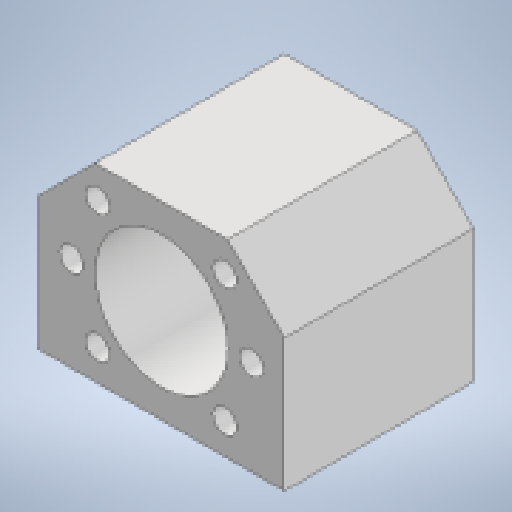
# Autodesk Inventor part: DSG16H
Saved by Autodesk Inventor 2023 (Build 270158000, 158)
## iProperties
Created: 2022-05-01
Part Number: DSG16H
Material: Generic
Document SubType Name: Modeling
Designer: plebbb
Density: 1 g/cm^3
Appearance: Default
Author: plebbb
Autodesk Inventor part; units mm, degrees
ref_plane "YZ Plane" through (0, 0, 0) normal (1, 0, 0) x (0, 1, 0)
ref_plane "XZ Plane" through (0, 0, 0) normal (0, 1, 0) x (-1, 0, 0)
ref_plane "XY Plane" through (0, 0, 0) normal (0, 0, 1) x (1, 0, 0)
sketch "Sketch1" plane through (0, 0, 0) normal (0, 0, 1) x (1, 0, 0)
  circle A0 centre (0, 0) radius 14
  line L0 (-26, -20) -> (26, -20)
  line L1 (26, -20) -> (26, 8)
  line L2 (26, 8) -> (14, 20)
  line L3 (14, 20) -> (-14, 20)
  line L4 (-14, 20) -> (-26, 8)
  line L5 (-26, 8) -> (-26, -20)
  circle A1 centre (0, 0) radius 19 construction
  circle A2 centre (13.435, 13.435) radius 2.5
  circle A3 centre (-13.435, -13.435) radius 2.5
  circle A4 centre (13.435, -13.435) radius 2.5
  circle A5 centre (-13.435, 13.435) radius 2.5
  circle A6 centre (-19, 0) radius 2.5
  circle A7 centre (19, 0) radius 2.5
  line L6 (-13.435, 13.435) -> (0, 0) construction
  line L7 (0, 0) -> (-19, 0) construction
  point P0 (0, 20)
  point P1 (0, -20)
  dimension "d0" = 28
  dimension "d1" = 40
  dimension "d2" = 52
  dimension "d3" = 38
  dimension "d4" = 5
  dimension "d5" = 45
  dimension "d6" = 20
  dimension "d7" = 135
  dimension "d8" = 12
  constraints: 16 end point, 8 centre point, 6 point on circle, 5 equal radius, 4 vertical alignment, 3 horizontal alignment, 3 perpendicular, 2 coincident, 2 equal length, 2 horizontal, 2 midpoint
  measures "d0" diameter of A0
  measures "d1" distance between parallel lines of L0 L3
  measures "d2" distance of L0.start L0.end
  measures "d3" diameter of A1
  measures "d4" diameter of A5
  measures "d5" angle of L6 L7
  measures "d6" distance from line of L0 A0.centre
  measures "d7" angle of L5 L4
  measures "d8" horizontal distance of L3.end L4.end
extrude "Extrusion1" add sketch "Sketch1" along normal blind 40
sketch "Sketch2" plane through (-26, -20, 0) normal (0, -1, 0) x (1, 0, 0)
  circle A0 centre (6, 32) radius 2.5
  circle A1 centre (46, 32) radius 2.5
  circle A2 centre (6, 8) radius 2.5
  circle A3 centre (46, 8) radius 2.5
  line L0 (6, 32) -> (46, 32) construction
  line L1 (46, 32) -> (46, 8) construction
  line L2 (46, 8) -> (6, 8) construction
  line L3 (6, 8) -> (6, 32) construction
  line L4 (0, 40) -> (52, 40) construction
  line L5 (52, 0) -> (52, 40) construction
  point P0 (26, 0)
  point P1 (26, 32)
  point P2 (26, 40)
  point P3 (46, 20)
  point P4 (52, 20)
  dimension "d11" = 5
  dimension "d12" = 40
  dimension "d13" = 24
  constraints: 8 end point, 4 centre point, 4 coincident, 4 midpoint, 3 equal radius, 2 parallel, 1 horizontal, 1 horizontal alignment, 1 perpendicular, 1 vertical alignment
  measures "d11" diameter of A1
  measures "d12" distance of L0.start L0.end
  measures "d13" distance of L0.end L1.end
extrude "Extrusion2" cut sketch "Sketch2" against normal blind 10
body "Solid1"
